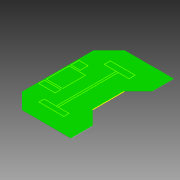
# Autodesk Inventor part: desk_clear_top
Saved by Autodesk Inventor 2015 (Build 190159000, 159)
## iProperties
Created: 2017-11-08
Part Number: desk_clear_top
Material: Generic
Document SubType Name: Modeling
Designer: windows7
Density: 1 g/cm^3
Appearance: Default
Author: windows7
Autodesk Inventor part; units mm, degrees
ref_plane "YZ Plane" through (0, 0, 0) normal (1, 0, 0) x (0, 1, 0)
ref_plane "XZ Plane" through (0, 0, 0) normal (0, 1, 0) x (-1, 0, 0)
ref_plane "Work Plane3" through (-2122.5168, 848.4088, -478.3521) normal (0, 0, 1) x (1, 0, 0)
sketch "Sketch1" plane through (-2122.5168, 848.4088, -478.3521) normal (0, 0, 1) x (1, 0, 0)
  line L0 (971.1279, -231.1279) -> (971.1279, 97.1564)
  line L1 (971.1279, 97.1564) -> (758.9959, 309.2884)
  line L2 (971.1279, 86.7336) -> (758.9959, 298.8657) projected
  line L3 (758.9959, 309.2884) -> (758.9959, 784.4356)
  line L4 (758.9959, 281.0041) -> (758.9959, 831.0041) projected
  line L5 (758.9959, 784.4356) -> (971.1279, 996.5676)
  line L6 (971.1279, 996.5676) -> (758.9959, 784.4356) projected
  line L7 (971.1279, 996.5676) -> (971.1279, 1324.8519)
  line L8 (971.1279, 1324.8519) -> (971.1279, 1024.8519) projected
  line L9 (971.1279, 1324.8519) -> (231.1279, 1324.8519)
  line L10 (231.1279, 1324.8519) -> (-6.862, 1086.862)
  line L11 (-6.862, 1086.862) -> (-5.362, 1088.362) projected
  line L12 (-6.862, 1086.862) -> (-6.862, 6.862)
  line L13 (-6.862, 6.862) -> (231.1279, -231.1279)
  line L14 (-3.7689, 3.7689) -> (-0.6658, 0.6658) projected
  line L15 (231.1279, -231.1279) -> (971.1279, -231.1279)
  point P0 (2122.5168, -848.4088)
  dimension "d2" = 740
  dimension "d3" = 1080
  dimension "d4" = 135
  dimension "d5" = 328.2843
  dimension "d6" = 328.2843
  dimension "d7" = 740
  dimension "d8" = 135
  dimension "d9" = 135
  dimension "d10" = 135
  dimension "d11" = 765.8579
  dimension "d12" = 977.9899
  dimension "d13" = 1555.9798
  constraints: 20 end point, 5 collinear, 3 parallel, 1 perpendicular, 1 vertical
  measures "d2" distance of L13.end L0.start
  measures "d3" distance of L10.end L12.end
  measures "d4" angle of L15 L13
  measures "d5" distance of L0.start L0.end
  measures "d6" distance of L5.end L7.end
  measures "d7" distance of L7.end L9.end
  measures "d8" angle of L9 L10
  measures "d9" angle of L7 L5
  measures "d10" angle of L0 L1
  measures "d11" distance between parallel lines of L12 L4
  measures "d12" horizontal distance of L7.end L10.end
  measures "d13" distance of L0.start L7.end
extrude "Extrusion1" add sketch "Sketch1" along normal blind 5
sketch "Sketch3" plane through (-2122.5168, 848.4088, -473.3521) normal (0, 0, 1) x (1, 0, 0)
  line L0 (9.5242, 357.2296) -> (9.5242, 702.0301)
  line L1 (9.5242, 702.0301) -> (255.8103, 702.0301)
  line L2 (255.8103, 702.0301) -> (255.8103, 357.2296)
  line L3 (255.8103, 357.2296) -> (9.5242, 357.2296)
  line L4 (254.1201, 1.9121) -> (629.6425, 1.9121)
  line L5 (629.6425, 1.9121) -> (629.6425, 80.2365)
  line L6 (629.6425, 80.2365) -> (254.1201, 80.2365)
  line L7 (254.1201, 80.2365) -> (254.1201, 1.9121)
  line L8 (254.1201, 986.5611) -> (629.6425, 986.5611)
  line L9 (629.6425, 986.5611) -> (629.6425, 1078.872)
  line L10 (629.6425, 1078.872) -> (254.1201, 1078.872)
  line L11 (254.1201, 1078.872) -> (254.1201, 986.5611)
  line L12 (435.9445, 80.2365) -> (466.7148, 80.2365)
  line L13 (466.7148, 80.2365) -> (466.7148, 986.5611)
  line L14 (466.7148, 986.5611) -> (435.9445, 986.5611)
  line L15 (435.9445, 986.5611) -> (435.9445, 80.2365)
  line L16 (758.9959, 309.2884) -> (758.9959, 784.4356) projected
  line L17 (10.8802, 243.43) -> (255.8103, 243.43)
  line L18 (255.8103, 243.43) -> (255.8103, 330.2134)
  line L19 (255.8103, 330.2134) -> (10.8802, 330.2134)
  line L20 (10.8802, 330.2134) -> (10.8802, 243.43)
  line L21 (10.8802, 727.5188) -> (149.2544, 727.5188)
  line L22 (149.2544, 727.5188) -> (149.2544, 848.202)
  line L23 (149.2544, 848.202) -> (10.8802, 848.202)
  line L24 (10.8802, 848.202) -> (10.8802, 727.5188)
  constraints: 48 end point, 10 parallel, 8 perpendicular, 5 horizontal, 5 point on line, 1 vertical
body "Solid1"
